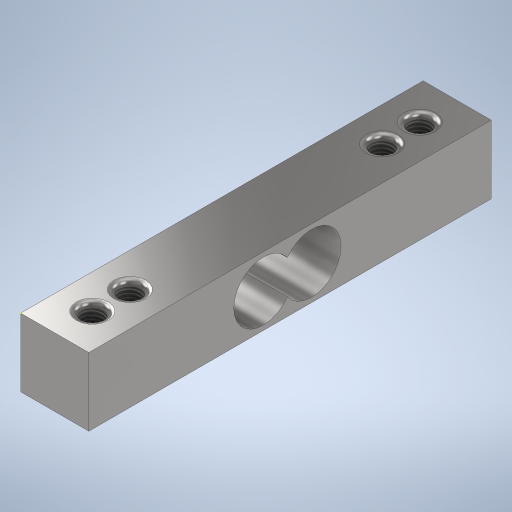
# Autodesk Inventor part: celula de carga
Saved by Autodesk Inventor 2023 (Build 270158000, 158)
## iProperties
Created: 2023-03-09
Part Number: celula de carga
Material: Iron, Malleable
Document SubType Name: Sheet Metal
Designer: Inteli
Density: 7.15 g/cm^3
Sheet Metal Rule: Padrão
Appearance: Semi-Polished
Author: Inteli
Autodesk Inventor part; units mm, degrees
ref_plane "YZ Plane" through (0, 0, 0) normal (1, 0, 0) x (0, 1, 0)
ref_plane "XZ Plane" through (0, 0, 0) normal (0, 1, 0) x (-1, 0, 0)
ref_plane "XY Plane" through (0, 0, 0) normal (0, 0, 1) x (1, 0, 0)
sketch "Sketch1" plane through (0, 0, 0) normal (0, 1, 0) x (-1, 0, 0)
  line L0 (0, 0) -> (0, -75)
  line L1 (0, -75) -> (-12.7, -75)
  line L2 (-12.7, -75) -> (-12.7, 0)
  line L3 (-12.7, 0) -> (0, 0)
  dimension "d0" = 75
  dimension "d1" = 12.7
  constraints: 8 end point, 3 perpendicular, 1 vertical
  measures "d0" distance of L0.start L0.end
  measures "d1" distance of L0.end L1.end
extrude "Extrusion1" add sketch "Sketch1" along normal blind 12.7
sketch "Sketch2" plane through (12.7, 0, 0) normal (1, 0, 0) x (0, 0, -1)
  line L0 (0, 0) -> (0, 12.7) projected
  arc A0 (37, 9.5123) -> (37, 3.1877) centre (32.5, 6.35) ccw
  arc A1 (37, 3.1877) -> (37, 9.5123) centre (41.5, 6.35) ccw
  line L1 (0, 0) -> (75, 0) projected
  line L2 (75, 0) -> (75, 12.7) projected
  line L3 (0, 12.7) -> (75, 12.7) projected
  line L4 (0, 0) -> (0, 12.7) projected
  dimension "d8" = 11
  constraints: 4 point on circle, 2 centre point
  measures "d8" diameter of A1
extrude "Extrusion2" cut sketch "Sketch2" against normal through all contours A1 A0
sketch "Sketch6" plane through (0, 12.7, 0) normal (0, 1, 0) x (1, 0, 0)
  line L0 (0, 0) -> (12.7, 0) projected
  circle A0 centre (6.35, 14) radius 2
  circle A1 centre (6.35, 7) radius 2
  line L1 (12.7, 75) -> (0, 75) projected
  circle A2 centre (6.35, 68) radius 2
  circle A3 centre (6.35, 61) radius 2
  dimension "d24" = 4
  dimension "d26" = 4
  dimension "d29" = 4
  constraints: 4 centre point
  measures "d24" diameter of A0
  measures "d26" diameter of A1
  measures "d29" diameter of A2
extrude "Extrusion5" cut sketch "Sketch6" against normal blind 5
sketch "Sketch7" plane through (0, 0, 0) normal (0, -1, 0) x (1, 0, 0)
  circle A0 centre (6.35, -14) radius 2 projected
  circle A1 centre (6.35, -14) radius 2
  circle A2 centre (6.35, -7) radius 2 projected
  circle A3 centre (6.35, -7) radius 2
  circle A4 centre (6.35, -68) radius 2 projected
  circle A5 centre (6.35, -68) radius 2
  circle A6 centre (6.35, -61) radius 2 projected
  circle A7 centre (6.35, -61) radius 2
  point P0 (0, 0)
  constraints: 4 centre point, 4 coincident
extrude "Extrusion6" cut sketch "Sketch7" against normal blind 5
fillet "Fillet1" radius 1 8 edges at (4.35, 0, -68) (4.35, 0, -61) (4.35, 0, -14) (4.35, 0, -7) (4.35, 12.7, -14) (4.35, 12.7, -7) (4.35, 12.7, -68) (4.35, 12.7, -61)
thread "Thread1" size "M4x0.7" class "6H" standard "ANSI Metric M Profile" full length
thread "Thread2" size "M4x0.7" class "6H" standard "ANSI Metric M Profile" full length
thread "Thread3" size "M4x0.7" class "6H" standard "ANSI Metric M Profile" full length
thread "Thread4" size "M4x0.7" class "6H" standard "ANSI Metric M Profile" full length
thread "Thread5" size "M4x0.7" class "6H" standard "ANSI Metric M Profile" full length
thread "Thread6" size "M4x0.7" class "6H" standard "ANSI Metric M Profile" full length
thread "Thread7" size "M4x0.7" class "6H" standard "ANSI Metric M Profile" full length
thread "Thread8" size "M4x0.7" class "6H" standard "ANSI Metric M Profile" full length
sketch "Esboço8" plane through (0, 12.7, 0) normal (0, 1, 0) x (1, 0, 0)
  point P0 (0, 0)
equation "\"BendRadius\" = Thickness"
equation "\"BendReliefWidth\" = Thickness"
equation "\"BendReliefDepth\" = 0.5 * Thickness"
equation "\"CornerReliefSize\" = 4 * Thickness"
equation "\"MinimumRemnant\" = 2 * Thickness"
equation "\"TransitionRadius\" = BendRadius"
equation "\"JacobiRadiusSize\" = BendRadius"
equation "\"GapSize\" = Thickness"
equation "\"Thickness\" = 3.048"
body "Solid1"
